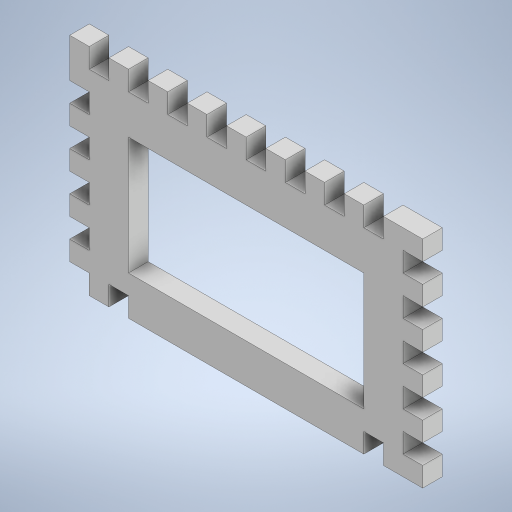
# Autodesk Inventor part: leftrightsidehole
Saved by Autodesk Inventor 2024 (Build 280153000, 153)
## iProperties
Created: 2024-04-16
Part Number: leftrightsidehole
Material: Generic
Document SubType Name: Modeling
Designer: srika
Density: 1 g/cm^3
Appearance: Default
Author: srika
Autodesk Inventor part; units mm, degrees
ref_plane "YZ Plane" through (0, 0, 0) normal (1, 0, 0) x (0, 1, 0)
ref_plane "XZ Plane" through (0, 0, 0) normal (0, 1, 0) x (-1, 0, 0)
ref_plane "XY Plane" through (0, 0, 0) normal (0, 0, 1) x (1, 0, 0)
sketch "Sketch1" plane through (0, 0, 0) normal (0, 0, 1) x (1, 0, 0)
  line L0 (5, 5) -> (85, 5)
  line L1 (85, 5) -> (85, 55)
  line L2 (85, 55) -> (5, 55)
  line L3 (5, 55) -> (5, 5)
  line L4 (0, 60) -> (5, 60)
  line L5 (5, 60) -> (5, 55)
  line L6 (5, 55) -> (0, 55)
  line L7 (0, 55) -> (0, 60)
  line L8 (0, 50) -> (5, 50)
  line L9 (5, 50) -> (5, 55)
  line L10 (5, 55) -> (0, 55)
  line L11 (0, 55) -> (0, 50)
  line L12 (5, 45) -> (0, 45)
  line L13 (0, 40) -> (5, 40)
  line L14 (5, 40) -> (5, 45)
  line L15 (5, 45) -> (0, 45)
  line L16 (0, 45) -> (0, 40)
  line L17 (5, 35) -> (0, 35)
  line L18 (0, 30) -> (5, 30)
  line L19 (5, 30) -> (5, 35)
  line L20 (5, 35) -> (0, 35)
  line L21 (0, 35) -> (0, 30)
  line L22 (5, 25) -> (0, 25)
  line L23 (0, 20) -> (5, 20)
  line L24 (5, 20) -> (5, 25)
  line L25 (5, 25) -> (0, 25)
  line L26 (0, 25) -> (0, 20)
  line L27 (5, 15) -> (0, 15)
  line L28 (0, 10) -> (5, 10)
  line L29 (5, 10) -> (5, 15)
  line L30 (5, 15) -> (0, 15)
  line L31 (0, 15) -> (0, 10)
  line L32 (15, 55) -> (10, 55)
  line L33 (15, 55) -> (10, 55)
  line L34 (10, 60) -> (15, 60)
  line L35 (10, 55) -> (10, 60)
  line L36 (15, 60) -> (15, 55)
  line L37 (25, 55) -> (20, 55)
  line L38 (25, 55) -> (20, 55)
  line L39 (20, 60) -> (25, 60)
  line L40 (20, 55) -> (20, 60)
  line L41 (25, 60) -> (25, 55)
  line L42 (35, 55) -> (30, 55)
  line L43 (35, 55) -> (30, 55)
  line L44 (30, 60) -> (35, 60)
  line L45 (30, 55) -> (30, 60)
  line L46 (35, 60) -> (35, 55)
  line L47 (45, 55) -> (40, 55)
  line L48 (45, 55) -> (40, 55)
  line L49 (40, 60) -> (45, 60)
  line L50 (40, 55) -> (40, 60)
  line L51 (45, 60) -> (45, 55)
  line L52 (55, 55) -> (50, 55)
  line L53 (55, 55) -> (50, 55)
  line L54 (50, 60) -> (55, 60)
  line L55 (50, 55) -> (50, 60)
  line L56 (55, 60) -> (55, 55)
  line L57 (65, 55) -> (60, 55)
  line L58 (65, 55) -> (60, 55)
  line L59 (60, 60) -> (65, 60)
  line L60 (60, 55) -> (60, 60)
  line L61 (65, 60) -> (65, 55)
  line L62 (75, 55) -> (70, 55)
  line L63 (75, 55) -> (70, 55)
  line L64 (70, 60) -> (75, 60)
  line L65 (70, 55) -> (70, 60)
  line L66 (75, 60) -> (75, 55)
  line L67 (85, 55) -> (80, 55)
  line L68 (85, 55) -> (80, 55)
  line L69 (80, 60) -> (85, 60)
  line L70 (80, 55) -> (80, 60)
  line L71 (85, 60) -> (85, 55)
  line L72 (90, 60) -> (85, 60)
  line L73 (85, 60) -> (85, 55)
  line L74 (85, 55) -> (90, 55)
  line L75 (90, 55) -> (90, 60)
  line L76 (90, 50) -> (85, 50)
  line L77 (85, 45) -> (90, 45)
  line L78 (90, 45) -> (90, 50)
  line L79 (90, 40) -> (85, 40)
  line L80 (85, 35) -> (90, 35)
  line L81 (90, 35) -> (90, 40)
  line L82 (90, 30) -> (85, 30)
  line L83 (85, 25) -> (90, 25)
  line L84 (90, 25) -> (90, 30)
  line L85 (90, 20) -> (85, 20)
  line L86 (85, 15) -> (90, 15)
  line L87 (90, 15) -> (90, 20)
  line L88 (90, 10) -> (85, 10)
  line L89 (85, 5) -> (90, 5)
  line L90 (90, 5) -> (90, 10)
  line L91 (10, 10) -> (15, 10)
  line L92 (15, 10) -> (15, 5)
  line L93 (15, 5) -> (10, 5)
  line L94 (10, 5) -> (10, 10)
  line L95 (75, 10) -> (80, 10)
  line L96 (80, 10) -> (80, 5)
  line L97 (80, 5) -> (75, 5)
  line L98 (75, 5) -> (75, 10)
  line L99 (15, 45) -> (75, 45)
  line L100 (75, 45) -> (75, 15)
  line L101 (75, 15) -> (15, 15)
  line L102 (15, 15) -> (15, 45)
  point P0 (0, 0)
  point P1 (10, 50)
  point P2 (20, 50)
  point P3 (30, 50)
  point P4 (40, 50)
  point P5 (50, 50)
  point P6 (60, 50)
  point P7 (70, 50)
  point P8 (80, 50)
  dimension "d2" = 10
  dimension "d9" = 10
  dimension "d16" = 10
  constraints: 206 end point, 14 parallel, 12 point on line, 8 horizontal, 7 perpendicular, 2 vertical, 163 other
  measures "d2" distance of L2.end L12.start
  measures "d9" distance of L2.end L32.start
  measures "d16" distance of L72.start L76.start
extrude "Extrusion1" add sketch "Sketch1" along normal blind 5 contours L3 L2 L1 L0 L96 L95 L98 L92 L91 L94 | L28 L31 L27 L3 | L23 L26 L22 L3 | L1 L88 L90 L89 | L18 L21 L17 L3 | L1 L85 L87 L86 | L13 L16 L12 L3 | L1 L82 L84 L83 | L8 L11 L6 L3 | L6 L7 L4 L5 | L1 L79 L81 L80 | L35 L34 L36 L2 | L1 L76 L78 L77 | L40 L39 L41 L2 | L2 L70 L69 L71 | L71 L72 L75 L74 | L45 L44 L46 L2 | L2 L65 L64 L66 | L50 L49 L51 L2 | L2 L60 L59 L61 | L55 L54 L56 L2
body "Solid1"
